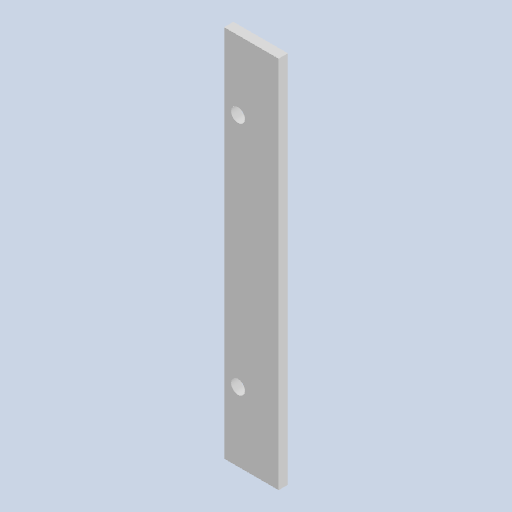
# Autodesk Inventor part: akkum_plate
Saved by Autodesk Inventor 2022 (Build 260153000, 153)
## iProperties
Created: 2024-07-28
Part Number: akkum_plate
Material: Типовые
Document SubType Name: Sheet Metal
Designer: Капустяник Андрей
Density: 1 g/cm^3
Sheet Metal Rule: По умолчанию
Appearance: По умолчанию
Author: Капустяник Андрей
Autodesk Inventor part; units mm, degrees
ref_plane "YZ Plane" through (0, 0, 0) normal (1, 0, 0) x (0, 1, 0)
ref_plane "XZ Plane" through (0, 0, 0) normal (0, 1, 0) x (-1, 0, 0)
ref_plane "XY Plane" through (0, 0, 0) normal (0, 0, 1) x (1, 0, 0)
sketch "Эскиз1" plane through (0, 0, 0) normal (0, 0, 1) x (1, 0, 0)
  line L0 (20.5, 40.5) -> (-20.5, 40.5)
  line L1 (-20.5, 40.5) -> (-20.5, -40.5)
  line L2 (-20.5, -40.5) -> (20.5, -40.5)
  line L3 (20.5, -40.5) -> (20.5, 40.5)
  line L4 (20.5, 40.5) -> (-20.5, -40.5) construction
  line L5 (-20.5, 40.5) -> (20.5, -40.5) construction
  line L6 (32.3, 42.5) -> (-32.3, 42.5)
  line L7 (-32.3, 42.5) -> (-32.3, -42.5)
  line L8 (-32.3, -42.5) -> (32.3, -42.5)
  line L9 (32.3, -42.5) -> (32.3, 42.5)
  line L10 (32.3, 42.5) -> (-32.3, -42.5) construction
  line L11 (-32.3, 42.5) -> (32.3, -42.5) construction
  line L12 (32.3, -42.5) -> (-32.3, -42.5)
  line L13 (-32.3, -42.5) -> (-32.3, 43.7)
  line L14 (-32.3, 43.7) -> (32.3, 43.7)
  line L15 (32.3, 43.7) -> (32.3, -42.5)
  line L16 (-20.5, -40.5) -> (-32.3, -40.5)
  line L17 (-32.3, -40.5) -> (-32.3, 40.5)
  line L18 (-32.3, 40.5) -> (-20.5, 40.5)
  line L19 (-20.5, 40.5) -> (-20.5, -40.5)
  point P0 (0, 0)
  dimension "d0" = 41
  dimension "d1" = 81
  dimension "d2" = 64.6
  dimension "d3" = 85
  dimension "d5" = 86.2
  measures "d0" distance of L2.end L1.end
  measures "d1" distance of L1.end L0.end
  measures "d2" distance of L8.end L7.end
  measures "d3" distance of L7.end L6.end
  measures "d5" distance between parallel lines of L8 L14
extrude "Пластина1" add sketch "Эскиз1" along normal blind 2 contours L1 L16 L7 L18
sketch "Эскиз2" plane through (0, 0, 0) normal (0, 0, -1) x (-1, 0, 0)
  circle A0 centre (29.3, 30.5) radius 1.45 projected
  circle A1 centre (29.3, -30.5) radius 1.45 projected
  circle A2 centre (29.3, 25.5) radius 1.6 projected
  circle A3 centre (29.3, -25.5) radius 1.6 projected
  circle A4 centre (29.3, 25.5) radius 1.5
  circle A5 centre (29.3, -25.5) radius 1.5
  point P0 (0, 0)
  dimension "d10" = 3
  dimension "d11" = 3
  constraints: 2 centre point, 2 coincident
  measures "d10" diameter of A4
  measures "d11" diameter of A5
extrude "Вырез1" cut sketch "Эскиз2" against normal blind 2 contours A4 | A5
equation "\"d8\" = Толщина"
equation "\"d4\" = Толщина"
equation "\"Радиус_гибки\" = Толщина"
equation "\"Ширина_просечки\" = Толщина"
equation "\"Глубина_просечки\" = 0.5 * Толщина"
equation "\"Размер_просечки\" = 4 * Толщина"
equation "\"Мин_остаток\" = 2 * Толщина"
equation "\"Радиус_перехода\" = Радиус_гибки"
equation "\"Радиус_Якоби\" = Радиус_гибки"
equation "\"Размер_зазора\" = Толщина"
equation "\"Толщина\" = 2"
